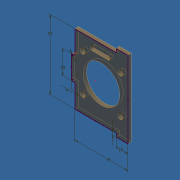
# Autodesk Inventor part: Fan_plate
Saved by Autodesk Inventor 2016 (Build 200138000, 138)
## iProperties
Created: 2016-04-03
Part Number: Fan_plate
Material: Polycarbonate, Smoke
Document SubType Name: Modeling
Designer: admin
Density: 1.2 g/cm^3
Appearance: Polycarbonate - Smoked
Author: admin
Autodesk Inventor part; units mm, degrees
ref_plane "YZ Plane" through (0, 0, 0) normal (1, 0, 0) x (0, 1, 0)
ref_plane "XZ Plane" through (0, 0, 0) normal (0, 1, 0) x (-1, 0, 0)
ref_plane "XY Plane" through (0, 0, 0) normal (0, 0, 1) x (1, 0, 0)
sketch "Sketch1" plane through (0, 0, 0) normal (0, 1, 0) x (-1, 0, 0)
  line L0 (17.5, -29.5) -> (-17.5, -29.5)
  line L1 (-17.5, -29.5) -> (-17.5, -32.5)
  line L2 (-17.5, -32.5) -> (-27.5, -32.5)
  line L3 (-27.5, -32.5) -> (-27.5, 32.5)
  line L4 (-27.5, 32.5) -> (-17.5, 32.5)
  line L5 (-17.5, 32.5) -> (-17.5, 29.5)
  line L6 (-17.5, 29.5) -> (17.5, 29.5)
  line L7 (17.5, -10) -> (19.5, -10)
  line L8 (20.5, -9) -> (20.5, 9)
  line L9 (19.5, 10) -> (17.5, 10)
  line L10 (17.5, 29.5) -> (17.5, 10)
  line L11 (17.5, -10) -> (17.5, -29.5)
  arc A0 (20.5, 9) -> (19.5, 10) centre (19.5, 9) ccw
  arc A1 (19.5, -10) -> (20.5, -9) centre (19.5, -9) ccw
  point P0 (0, 0)
  point P1 (-27.5, 0)
  point P2 (0, -29.5)
  point P3 (20.5, 0)
  dimension "d19" = 59
  dimension "d20" = 45
  dimension "d21" = 10
  dimension "d22" = 3
  dimension "d23" = 20
  dimension "d26" = 2
  dimension "d27" = 3
  constraints: 24 end point, 5 perpendicular, 4 horizontal, 4 point on circle, 4 tangent, 3 collinear, 3 midpoint, 2 centre point, 2 horizontal alignment, 2 vertical, 1 equal radius, 1 point on line, 1 vertical alignment
  measures "d19" distance between parallel lines of L6 L0
  measures "d20" distance between parallel lines of L3 L11
  measures "d21" distance of L1.end L2.end
  measures "d22" distance of L0.end L1.end
  measures "d23" distance of L7.end L9.start
  measures "d26" diameter of A0
  measures "d27" distance between parallel lines of L11 L8
extrude "Extrusion1" add sketch "Sketch1" along normal blind 3
sketch "Sketch2" plane through (0, 3, 0) normal (0, 1, 0) x (1, 0, 0)
  line L0 (-11, 16) -> (21, 16) construction
  line L1 (-17.5, 29.5) -> (-17.5, 10) projected
  line L2 (27.5, -32.5) -> (27.5, 32.5) projected
  line L3 (-17.5, 25.7242) -> (27.5, 25.7242) construction
  point P0 (0, 0)
  point P1 (-11, -16)
  point P2 (21, -16)
  point P3 (5, 25.7242)
  point P4 (5, 16)
  dimension "d7" = 32
  dimension "d8" = 32
  dimension "d10" = 16
  constraints: 4 end point, 3 vertical alignment, 2 horizontal alignment, 2 midpoint, 2 point on line, 1 horizontal, 1 perpendicular
  measures "d7" distance of L0.start L0.end
  measures "d8" distance of point (21, -16) L0.end
  measures "d10" vertical distance of point (0, 0) point (21, -16)
hole "Hole1" at (-11, 3, 16) at (-11, 3, -16) at (21, 3, 16) at (21, 3, -16) direction (0, -1, 0) diameter 4 end through all
sketch "Sketch3" plane through (0, 3, 0) normal (0, 1, 0) x (1, 0, 0)
  circle A0 centre (21, -16) radius 2 projected
  circle A1 centre (-11, -16) radius 2 projected
  circle A2 centre (-11, 16) radius 2 projected
  circle A3 centre (21, 16) radius 2 projected
  line L0 (17.5, 29.5) -> (-17.5, 29.5) projected
  line L1 (-17.5, 29.5) -> (-17.5, 10) projected
  line L2 (-17.5, 10) -> (-19.5, 10) projected
  line L3 (-20.5, 9) -> (-20.5, -9) projected
  line L4 (-19.5, -10) -> (-17.5, -10) projected
  line L5 (-17.5, -10) -> (-17.5, -29.5) projected
  line L6 (-17.5, -29.5) -> (17.5, -29.5) projected
  line L7 (17.5, -29.5) -> (17.5, -32.5) projected
  line L8 (17.5, -32.5) -> (27.5, -32.5) projected
  line L9 (27.5, -32.5) -> (27.5, 32.5) projected
  line L10 (27.5, 32.5) -> (17.5, 32.5) projected
  line L11 (17.5, 32.5) -> (17.5, 29.5) projected
  line L12 (-11, 16) -> (21, -16) construction
  line L13 (-11, -16) -> (21, 16) construction
  circle A4 centre (5, 0) radius 15.5278
  arc A5 (-19.5, 10) -> (-20.5, 9) centre (-19.5, 9) ccw projected
  arc A6 (-20.5, -9) -> (-19.5, -10) centre (-19.5, -9) ccw projected
  line L14 (-2.9348, -23.5081) -> (10.6481, -23.5081)
  line L15 (10.6481, -20.5081) -> (-2.9348, -20.5081)
  arc A7 (-2.9348, -20.5081) -> (-2.9348, -23.5081) centre (-2.9348, -22.0081) ccw
  arc A8 (10.6481, -23.5081) -> (10.6481, -20.5081) centre (10.6481, -22.0081) ccw
  point P0 (0, 0)
  dimension "d28" = 3
  constraints: 8 end point, 4 point on circle, 4 tangent, 3 centre point, 1 horizontal, 1 midpoint, 1 parallel, 1 perpendicular
  measures "d28" distance between parallel lines of L14 L15
extrude "Extrusion2" cut sketch "Sketch3" against normal up to next contours A4 | A7 L15 A8 L14
equation "\"d27\" = d22"
equation "\"d8\" = d7"
equation "\"d10\" = d9"
equation "\"d9\" = 0.5 * d7"
body "Solid1"
